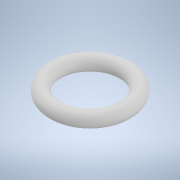
# Autodesk Inventor part: oring
Saved by Autodesk Inventor 2022 (Build 260153000, 153)
## iProperties
Created: 2022-01-05
Part Number: oring
Material: Genérico
Document SubType Name: Modeling
Designer: JK
Density: 1 g/cm^3
Appearance: Valor por defecto
Author: JK
Autodesk Inventor part; units mm, degrees
ref_plane "YZ Plane" through (0, 0, 0) normal (1, 0, 0) x (0, 1, 0)
ref_plane "XZ Plane" through (0, 0, 0) normal (0, 1, 0) x (-1, 0, 0)
ref_plane "XY Plane" through (0, 0, 0) normal (0, 0, 1) x (1, 0, 0)
sketch "Boceto1" plane through (0, 0, 0) normal (0, 1, 0) x (-1, 0, 0)
  circle A0 centre (0, 0) radius 6.125
  dimension "d0" = 12.25
  constraints: 1 centre point, 1 coincident
  measures "d0" diameter of A0
sketch "Boceto2" plane through (0, 0, 0) normal (1, 0, 0) x (0, 1, 0)
  circle A0 centre (0, 6.125) radius 1.25
  line L0 (0, -6.125) -> (0, 6.125) projected
  point P0 (0, 0)
  dimension "d1" = 2.5
  constraints: 1 centre point, 1 coincident
  measures "d1" diameter of A0
sweep "Barrido1" add profiles "Boceto2" path "Boceto1"
